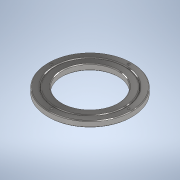
# Autodesk Inventor part: lazy_susan
Saved by Autodesk Inventor 2021 (Build 250183000, 183)
## iProperties
Created: 2021-04-04
Part Number: lazy_susan
Material: Generic
Document SubType Name: Modeling
Designer: jorge
Density: 1 g/cm^3
Appearance: Steel - Polished
Author: jorge
Autodesk Inventor part; units mm, degrees
ref_plane "YZ Plane" through (0, 0, 0) normal (1, 0, 0) x (0, 1, 0)
ref_plane "XZ Plane" through (0, 0, 0) normal (0, 1, 0) x (-1, 0, 0)
ref_plane "XY Plane" through (0, 0, 0) normal (0, 0, 1) x (1, 0, 0)
sketch "Sketch1" plane through (0, 0, 0) normal (0, 1, 0) x (-1, 0, 0)
  circle A0 centre (0, 0) radius 39.9
  circle A1 centre (0, 0) radius 50
  circle A2 centre (0, 0) radius 60
  circle A3 centre (0, 0) radius 50.5
  dimension "d0" = 79.8
  dimension "d1" = 100
  dimension "d2" = 120
  dimension "d3" = 101
  constraints: 4 centre point, 4 coincident
  measures "d0" diameter of A0
  measures "d1" diameter of A1
  measures "d2" diameter of A2
  measures "d3" diameter of A3
extrude "Extrusion1" add sketch "Sketch1" along normal blind 8.5
chamfer "Chamfer1" distance 1 angle 45 4 edges at (60, 8.5, 0) (60, 0, 0) (39.9, 8.5, 0) (39.9, 0, 0)
chamfer "Chamfer2" distance 1 angle 45 4 edges at (50.5, 8.5, 0) (50, 8.5, 0) (50.5, 0, 0) (50, 0, 0)
sketch "Sketch2" plane through (0, 8.5, 0) normal (0, 1, 0) x (1, 0, 0)
  circle A0 centre (0, 55.0004) radius 1.6
  circle A1 centre (-55, 0) radius 1.6
  circle A2 centre (0, -55.0004) radius 1.6
  circle A3 centre (55, 0) radius 1.6
  circle A4 centre (0, 0) radius 59 projected
  circle A5 centre (0, 0) radius 51.5 projected
  dimension "d12" = 3.2
  dimension "d13" = 3.2
  dimension "d14" = 3.2
  dimension "d15" = 3.2
  dimension "d16" = 77.782
  dimension "d17" = 77.782
  dimension "d18" = 77.782
  dimension "d19" = 77.782
  dimension "d20" = 0
  dimension "d21" = 0
  dimension "d22" = 0
  dimension "d25" = 55
  constraints: 4 centre point
  measures "d12" diameter of A0
  measures "d13" diameter of A1
  measures "d14" diameter of A2
  measures "d15" diameter of A3
  measures "d16" distance of A2.centre A3.centre
  measures "d17" distance of A0.centre A3.centre
  measures "d18" distance of A1.centre A2.centre
  measures "d19" distance of A1.centre A0.centre
  measures "d20" vertical distance of A1.centre point (0, 0)
  measures "d21" horizontal distance of point (0, 0) A0.centre
  measures "d22" vertical distance of point (0, 0) A3.centre
  measures "d25" distance of point (0, 0) A1.centre
extrude "Extrusion2" cut sketch "Sketch2" against normal up to surface (8.5 mm away) contours A0 | A1 | A2 | A3
body "Solid1"
